3.2mm_thickwall (Autodesk Fusion 360 design; units mm, degrees)
Autodesk Fusion 360 part; units mm, degrees
sketch "Sketch1" plane through (0, 0, 0) normal (0, 1, 0) x (1, 0, 0)
  line L0 (0, 0) -> (0, -1.4)
  line L1 (0, -1.4) -> (0.1, -1.5)
  line L2 (0.1, -1.5) -> (0.5, -1.5)
  line L3 (0.5, -1.5) -> (0.5, 0)
  line L4 (0.5, 0) -> (0, 0)
  line L5 (0, -1.29) -> (-0.25, -1.29)
  line L6 (-0.25, -1.29) -> (-0.25, -1.24)
  line L7 (-0.25, -1.24) -> (-0.95, -1.24)
  line L8 (-0.95, -1.24) -> (-0.95, -1.29)
  line L9 (-0.95, -1.29) -> (-2.4, -1.29)
  line L10 (-2.4, -1.29) -> (-3, -1.14)
  line L11 (-3, -1.14) -> (-3, -0.915)
  line L12 (-3, -0.915) -> (0, -0.915)
  dimension "d2" = 0.1
  dimension "d3" = 0.1
  dimension "d4" = 0.4
  dimension "d5" = 0.915
  dimension "d7" = 0.25
  dimension "d8" = 0.7
  dimension "d10" = 0.6
  dimension "d11" = 0.15
  dimension "d12" = 3
  dimension "d27" = 1.5
  dimension "d28" = 1.29
  dimension "d29" = 0.05
  constraint coincident L0.start L4.end
  constraint vertical L0
  constraint perpendicular L0 L2
  constraint perpendicular L2 L3
  constraint perpendicular L0 L4
  constraint coincident L0 L5.start
  constraint perpendicular L0 L5
  constraint perpendicular L5 L6
  constraint perpendicular L0 L7
  constraint perpendicular L7 L8
  constraint perpendicular L8 L9
  constraint perpendicular L9 L11
  constraint perpendicular L8 L12
  constraint collinear L5 L9
  measures "d2" horizontal distance of L0.end L1.end
  measures "d3" vertical distance of L0.end L1.end
  measures "d4" distance of L1.end L2.end
  measures "d5" distance of L0.start L12
  measures "d7" distance of L5.start L5.end
  measures "d8" distance of L6.end L7.end
  measures "d10" horizontal distance of L9.end L10.end
  measures "d11" vertical distance of L9.end L10.end
  measures "d12" distance of L0 L11
  measures "d27" distance of L2 L4
  measures "d28" distance of L0.start L9
  measures "d29" distance of L7.end L8.end
revolve "Revolve1" add sketch "Sketch1" angle 360 about axis through (0.5, 0, 0) along (-1, 0, 0)
sketch "Sketch3" plane through (0.5, 0, 0) normal (1, 0, 0) x (0, 1, 0)
  circle A0 centre (0, 0) radius 1.5
  arc A1 (-0.9236, -1.1839) -> (-0.7144, -1.2438) centre (-0.7441, -0.9516) ccw
  line L0 (-1.4035, 0.2951) -> (-1.3135, 0.0926)
  arc A2 (0.7991, -0.077) -> (1.4755, 0.2779) centre (1.1676, 0.0428) cw
  line L1 (-0.153, 1.4257) -> (-0.3178, 1.2775)
  arc A3 (-1.3135, 0.0926) -> (-1.2191, -0.0246) centre (-1.0496, 0.2086) ccw
  arc A4 (0.0514, 1.5003) -> (-0.153, 1.4257) centre (0.0427, 1.2068) ccw
  arc A5 (1.4755, 0.2779) -> (1.4431, 0.4144) centre (0.0001, -0.0005) ccw
  arc A6 (-0.6015, 0.5316) -> (-1.3573, 0.642) centre (-0.97, 0.6513) cw
  line L2 (0.9719, 0.736) -> (0.32, 0.736)
  line L3 (0.9619, -1.0641) -> (1.0081, -0.8474)
  arc A7 (-1.3573, 0.642) -> (-1.4113, 0.5125) centre (0, 0) ccw
  arc A8 (-1.4113, 0.5125) -> (-1.4035, 0.2951) centre (-1.1348, 0.4135) ccw
  line L4 (-0.3534, -1.1672) -> (0.174, -0.784)
  arc A9 (1.0081, -0.8474) -> (1.0006, -0.6971) centre (0.7264, -0.7861) ccw
  arc A10 (-0.6915, -0.4079) -> (-1.0301, -1.0926) centre (-0.9192, -0.7214) cw
  arc A11 (0.8403, -1.2445) -> (0.9619, -1.0641) centre (0.6749, -1.002) ccw
  arc A12 (1.1172, 0.6967) -> (0.9719, 0.736) centre (0.9719, 0.4477) ccw
  arc A13 (0.7205, -1.3176) -> (0.8403, -1.2445) centre (-0.0002, -0.0004) ccw
  arc A14 (-1.0301, -1.0926) -> (-0.9236, -1.1839) centre (-0.0001, -0.0001) ccw
  arc A15 (1.4431, 0.4144) -> (1.309, 0.5858) centre (1.1612, 0.332) ccw
  arc A16 (0.32, 0.736) -> (0.1913, 1.4889) centre (0.3197, 1.1234) cw
  line L5 (1.0006, -0.6971) -> (0.7991, -0.077)
  arc A17 (-0.3178, 1.2775) -> (-0.4, 1.1515) centre (-0.1259, 1.0624) ccw
  line L6 (-0.7144, -1.2438) -> (-0.4941, -1.2208)
  line L7 (1.309, 0.5858) -> (1.1172, 0.6967)
  line L8 (-1.2191, -0.0246) -> (-0.6915, -0.4079)
  arc A18 (0.174, -0.784) -> (0.7205, -1.3176) centre (0.4017, -1.0974) cw
  line L9 (-0.4, 1.1515) -> (-0.6015, 0.5316)
  arc A19 (-0.4941, -1.2208) -> (-0.3534, -1.1672) centre (-0.5229, -0.9339) ccw
  arc A20 (0.1913, 1.4889) -> (0.0514, 1.5003) centre (0.0001, -0.0003) ccw
  circle A21 centre (0, 0) radius 1.5012
  constraint coincident A0.centre A7.centre
  constraint coincident A16.end A21
extrude "Extrude2" add sketch "Sketch3" along normal blind 1 contours A0 A1 L0 A2 L1 A3 A4 A6 L2 L3 A8 L4 A9 A10 A11 A12 A15 A16 L5 A17 L6 L7 L8 A18 L9 A19 | A0 A2 A15 A21 | A0 A11 A18 A21 | A2 A5 A15 A21 | A0 A4 A16 A20 A21 | A0 A1 A10 A21 | A1 A10 A14 A21 | A0 A6 A8 A21 | A7 A8 A21
move_body "Move1" bodies 1 to x (0, 0, 1) y (0, 1, 0) z (-1, 0, 0) at (0, 0, 0)
equation "d5 = ( 1.83 / 2 ) * 1 mm"
equation "d27 = 3 mm / 2"
equation "d28 = var / 2"
equation "var = 2.580 mm"
